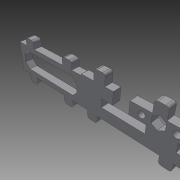
# Autodesk Inventor part: x_iddler_wall_lower
Saved by Autodesk Inventor 2014 (Build 180170000, 170)
## iProperties
Created: 2013-12-02
Part Number: x_iddler_wall_lower
Material: Generic
Document SubType Name: Modeling
Designer: buben
Density: 1 g/cm^3
Appearance: Default
Author: buben
Subject: Laser Cutted
Autodesk Inventor part; units mm, degrees
ref_plane "YZ Plane" through (0, 0, 0) normal (1, 0, 0) x (0, 1, 0)
ref_plane "XZ Plane" through (0, 0, 0) normal (0, 1, 0) x (-1, 0, 0)
ref_plane "XY Plane" through (0, 0, 0) normal (0, 0, 1) x (1, 0, 0)
sketch "Sketch1" plane through (0, 0, 0) normal (0, 1, 0) x (-1, 0, 0)
  line L0 (0, 0) -> (128, 0)
  line L1 (128, 0) -> (128, 22)
  line L2 (52, 14) -> (52, 8)
  line L3 (52, 8) -> (22, 8)
  line L4 (22, 8) -> (22, 14)
  circle A0 centre (5.5, 18.5) radius 2.25
  circle A1 centre (5.5, 18.5) radius 4.5 construction
  circle A2 centre (25.5, 18.5) radius 2.25
  circle A3 centre (25.5, 18.5) radius 4.5 construction
  line L5 (33, 14) -> (44, 14) construction
  circle A4 centre (38.5, 19.099) radius 7.5 construction
  circle A5 centre (38.5, 19.099) radius 4 construction
  line L6 (33, 23) -> (33, 14)
  line L7 (44, 14) -> (44, 23)
  line L8 (22, 14) -> (33, 14)
  line L9 (44, 14) -> (52, 14)
  line L10 (0, 14) -> (4, 14)
  line L11 (4, 14) -> (4, 8)
  line L12 (4, 8) -> (0, 8)
  line L13 (0, 23) -> (0, 14)
  line L14 (0, 8) -> (0, 0)
  line L15 (11.5, 23) -> (11.5, 29)
  line L16 (13.5, 31) -> (17.5, 31)
  line L17 (19.5, 29) -> (19.5, 23)
  arc A6 (13.5, 31) -> (11.5, 29) centre (13.5, 29) ccw
  arc A7 (19.5, 29) -> (17.5, 31) centre (17.5, 29) ccw
  line L18 (33, 23) -> (19.5, 23)
  line L19 (11.5, 23) -> (0, 23)
  line L20 (50, 23) -> (50, 29)
  line L21 (52, 31) -> (56, 31)
  line L22 (58, 29) -> (58, 23)
  arc A8 (52, 31) -> (50, 29) centre (52, 29) ccw
  arc A9 (58, 29) -> (56, 31) centre (56, 29) ccw
  line L23 (68, 23) -> (58, 23)
  line L24 (50, 23) -> (44, 23)
  line L25 (68, 23) -> (68, 22)
  line L26 (68, 22) -> (128, 22)
  line L27 (19.5, 16.7896) -> (15.5, 14.4802)
  line L28 (15.5, 14.4802) -> (11.5, 16.7896)
  line L29 (11.5, 16.7896) -> (11.5, 21.4084)
  line L30 (11.5, 21.4084) -> (15.5, 23.7178)
  line L31 (15.5, 23.7178) -> (19.5, 21.4084)
  line L32 (19.5, 21.4084) -> (19.5, 16.7896)
  point P0 (15.5, 19.099)
  point P1 (0, 18.5)
  point P2 (15.5, 31)
  point P3 (15.5, 19.099)
  dimension "d0" = 6
  dimension "d1" = 8
  dimension "d3" = 4.5
  dimension "d4" = 9
  dimension "d5" = 4.5
  dimension "d6" = 9
  dimension "d8" = 11
  dimension "d9" = 8
  dimension "d10" = 15
  dimension "d11" = 9
  dimension "d12" = 4
  dimension "d13" = 5.5
  dimension "d14" = 10
  dimension "d15" = 10
  dimension "d16" = 2
  dimension "d17" = 8
  dimension "d18" = 8
  dimension "d19" = 23
  dimension "d20" = 30
  dimension "d21" = 18
  dimension "d23" = 2
  dimension "d24" = 8
  dimension "d25" = 6
  dimension "d26" = 8
  dimension "d27" = 10
  dimension "d29" = 60
  dimension "d30" = 8
  constraints: 66 end point, 18 perpendicular, 11 parallel, 10 centre point, 10 collinear, 10 point on circle, 8 tangent, 4 coincident, 4 horizontal alignment, 3 horizontal, 2 equal radius, 2 midpoint, 1 vertical alignment, 13 other
  measures "d0" distance of L3.end L4.end
  measures "d1" distance between parallel lines of L0 L3
  measures "d3" diameter of A0
  measures "d4" diameter of A1
  measures "d5" diameter of A2
  measures "d6" diameter of A3
  measures "d8" distance of L5.start L5.end
  measures "d9" diameter of A5
  measures "d10" diameter of A4
  measures "d11" distance of L5.end L7.end
  measures "d12" distance of L10.start L10.end
  measures "d13" distance from line of A0.centre L13
  measures "d14" horizontal distance of A0.centre point (15.5, 19.099)
  measures "d15" horizontal distance of A2.centre point (15.5, 19.099)
  measures "d16" radius of A6
  measures "d17" distance between parallel lines of L17 L15
  measures "d18" distance between parallel lines of L19 L16
  measures "d19" distance of A4.centre point (15.5, 19.099)
  measures "d20" distance of L2.end L3.end
  measures "d21" distance between parallel lines of L4 L11
  measures "d23" radius of A8
  measures "d24" distance between parallel lines of L22 L20
  measures "d25" distance between parallel lines of L20 L7
  measures "d26" distance between parallel lines of L9 L26
  measures "d27" distance between parallel lines of L22 L25
  measures "d29" distance of L25.end L1.end
  measures "d30" distance between parallel lines of L32 L29
extrude "Extrusion1" add sketch "Sketch1" along normal blind 6
sketch "Sketch2" plane through (0, 6, 0) normal (0, 1, 0) x (1, 0, 0)
  line L0 (-128, 0) -> (-128, -22) projected
  line L1 (-128, -22) -> (-68, -22) projected
  line L2 (-68, -22) -> (-68, -23) projected
  line L3 (-120, -22) -> (-112, -22)
  line L4 (-112, -22) -> (-112, -26)
  line L5 (-114, -28) -> (-118, -28)
  line L6 (-120, -26) -> (-120, -22)
  line L7 (-84, -22) -> (-76, -22)
  line L8 (-76, -22) -> (-76, -26)
  line L9 (-78, -28) -> (-82, -28)
  line L10 (-84, -26) -> (-84, -22)
  arc A0 (-84, -26) -> (-82, -28) centre (-82, -26) ccw
  arc A1 (-78, -28) -> (-76, -26) centre (-78, -26) ccw
  arc A2 (-114, -28) -> (-112, -26) centre (-114, -26) ccw
  arc A3 (-120, -26) -> (-118, -28) centre (-118, -26) ccw
  dimension "d33" = 2
  dimension "d34" = 8
  dimension "d35" = 6
  dimension "d36" = 8
  dimension "d37" = 8
  dimension "d38" = 8
  constraints: 16 end point, 8 point on circle, 8 tangent, 4 centre point, 4 parallel, 3 equal radius, 2 horizontal, 2 perpendicular, 2 point on line, 1 collinear
  measures "d33" radius of A0
  measures "d34" distance between parallel lines of L8 L10
  measures "d35" distance between parallel lines of L1 L9
  measures "d36" distance between parallel lines of L4 L6
  measures "d37" distance between parallel lines of L2 L8
  measures "d38" distance between parallel lines of L0 L6
extrude "Extrusion2" add sketch "Sketch2" against normal blind 6
sketch "Sketch3" plane through (0, 6, 0) normal (0, 1, 0) x (1, 0, 0)
  line L0 (0, 0) -> (-128, 0) projected
  line L1 (-112, -26) -> (-112, -22) projected
  line L2 (-76, -26) -> (-76, -22) projected
  line L3 (0, -8) -> (0, 0) projected
  line L4 (-120, 0) -> (-112, 0)
  line L5 (-112, 0) -> (-112, 4)
  line L6 (-114, 6) -> (-118, 6)
  line L7 (-120, 4) -> (-120, 0)
  line L8 (-84, 0) -> (-76, 0)
  line L9 (-76, 0) -> (-76, 4)
  line L10 (-78, 6) -> (-82, 6)
  line L11 (-84, 4) -> (-84, 0)
  line L12 (-63, 0) -> (-55, 0)
  line L13 (-55, 0) -> (-55, 4)
  line L14 (-57, 6) -> (-61, 6)
  line L15 (-63, 4) -> (-63, 0)
  line L16 (-12, 0) -> (-4, 0)
  line L17 (-4, 0) -> (-4, 4)
  line L18 (-6, 6) -> (-10, 6)
  line L19 (-12, 4) -> (-12, 0)
  arc A0 (-118, 6) -> (-120, 4) centre (-118, 4) ccw
  arc A1 (-112, 4) -> (-114, 6) centre (-114, 4) ccw
  arc A2 (-82, 6) -> (-84, 4) centre (-82, 4) ccw
  arc A3 (-76, 4) -> (-78, 6) centre (-78, 4) ccw
  arc A4 (-61, 6) -> (-63, 4) centre (-61, 4) ccw
  arc A5 (-55, 4) -> (-57, 6) centre (-57, 4) ccw
  arc A6 (-10, 6) -> (-12, 4) centre (-10, 4) ccw
  arc A7 (-4, 4) -> (-6, 6) centre (-6, 4) ccw
  dimension "d41" = 2
  dimension "d42" = 6
  dimension "d43" = 8
  dimension "d44" = 8
  dimension "d45" = 8
  dimension "d46" = 8
  dimension "d47" = 4
  dimension "d48" = 43
  constraints: 32 end point, 16 point on circle, 16 tangent, 8 centre point, 8 parallel, 7 equal radius, 5 collinear, 4 horizontal, 4 perpendicular, 4 point on line
  measures "d41" radius of A0
  measures "d42" distance between parallel lines of L0 L6
  measures "d43" distance between parallel lines of L5 L7
  measures "d44" distance between parallel lines of L9 L11
  measures "d45" distance between parallel lines of L13 L15
  measures "d46" distance between parallel lines of L17 L19
  measures "d47" distance between parallel lines of L3 L17
  measures "d48" distance between parallel lines of L19 L13
extrude "Extrusion3" add sketch "Sketch3" against normal blind 6
sketch "Sketch4" plane through (0, 0, 0) normal (0, -1, 0) x (1, 0, 0)
  line L0 (-112, 22) -> (-84, 22) projected
  line L1 (-128, 0) -> (-128, 22) projected
  line L2 (-84, 0) -> (-112, 0) projected
  line L3 (-63, 0) -> (-76, 0) projected
  line L4 (-4, -4) -> (-4, 0) projected
  line L5 (-124, 14) -> (-124, 8)
  line L6 (-124, 8) -> (-120, 4)
  line L7 (-120, 4) -> (-76, 4)
  line L8 (-76, 4) -> (-72, 8)
  line L9 (-72, 8) -> (-72, 14)
  line L10 (-72, 14) -> (-76, 18)
  line L11 (-76, 18) -> (-120, 18)
  line L12 (-120, 18) -> (-124, 14)
  line L13 (-68, 22) -> (-68, 0) construction
  dimension "d52" = 45
  dimension "d53" = 4
  dimension "d54" = 4
  dimension "d55" = 4
  dimension "d56" = 4
  dimension "d57" = 4
  constraints: 18 end point, 8 perpendicular, 3 parallel, 1 point on line
  measures "d52" angle of L6 L5
  measures "d53" distance between parallel lines of L0 L11
  measures "d54" distance between parallel lines of L2 L7
  measures "d55" distance between parallel lines of L1 L5
  measures "d56" distance between parallel lines of L13 L9
  measures "d57" horizontal distance of L11.end L5.start
extrude "Extrusion4" cut sketch "Sketch4" against normal blind 6
body "Solid1"
